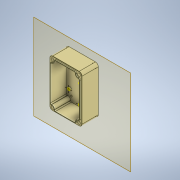
# Autodesk Inventor part: PinfoxBox
Saved by Autodesk Inventor 2021 (Build 250183000, 183)
## iProperties
Created: 2021-02-15
Part Number: PinfoxBox
Material: Polypropylene
Document SubType Name: Modeling
Designer: James
Density: 0.899 g/cm^3
Appearance: Smooth - Ash
Author: James
Autodesk Inventor part; units mm, degrees
ref_plane "YZ Plane" through (0, 0, 0) normal (1, 0, 0) x (0, 1, 0)
ref_plane "XZ Plane" through (0, 0, 0) normal (0, 1, 0) x (-1, 0, 0)
ref_plane "XY Plane" through (0, 0, 0) normal (0, 0, 1) x (1, 0, 0)
sketch "Drawing" plane through (0, 0, 0) normal (0, 0, 1) x (1, 0, 0)
  line L0 (-58.5227, 93.5052) -> (128.141, 93.5052) construction
  line L1 (128.141, 93.5052) -> (128.141, -71.3811) construction
  line L2 (128.141, -71.3811) -> (-58.5227, -71.3811) construction
  line L3 (-58.5227, -71.3811) -> (-58.5227, 93.5052) construction
  line L4 (-58.5227, 93.5052) -> (-58.5227, 50)
  line L5 (-54.9683, 50) -> (-54.9683, -50)
  line L6 (-58.5227, 50) -> (-54.9683, 50)
  line L7 (0, 0) -> (-54.9683, 0) construction
  line L8 (0, 0) -> (0, 93.5052) construction
  line L9 (0, 93.5052) -> (0, -71.3811)
  line L10 (-58.5227, 0) -> (128.141, 0)
  circle A0 centre (23, 22.25) radius 2.5
  circle A1 centre (23, 22.25) radius 1.5
  circle A2 centre (20, 35) radius 1.75
  dimension "d16" = 164.8863
  dimension "d20" = 3.5544
  dimension "d21" = 100
  dimension "d22" = 43.5052
  dimension "d48" = 5
  dimension "d49" = 1
  dimension "d50" = 3.5
  constraints: 14 end point, 5 point on line, 4 perpendicular, 3 centre point, 3 coincident, 1 horizontal, 1 midpoint, 1 vertical, 2 other
  measures "d16" distance of L2.end L0.start
  measures "d20" distance of L4.end L5.start
  measures "d21" distance of L5.start L5.end
  measures "d22" distance of L4.start L4.end
  measures "d48" diameter of A0
  measures "d49" radial gap between concentric circles of A0 A1
  measures "d50" diameter of A2
sketch "Sketch2" plane through (0, 0, 0) normal (0, 0, 1) x (1, 0, 0)
  line L0 (28, 50) -> (-28, 50)
  line L1 (-34, 44) -> (-34, -44)
  line L2 (-28, -50) -> (28, -50)
  line L3 (34, -44) -> (34, 44)
  line L4 (34, 50) -> (-34, -50) construction
  line L5 (-34, 50) -> (34, -50) construction
  arc A0 (-28, 50) -> (-34, 44) centre (-28, 44) ccw
  arc A1 (34, 44) -> (28, 50) centre (28, 44) ccw
  arc A2 (-34, -44) -> (-28, -50) centre (-28, -44) ccw
  arc A3 (28, -50) -> (34, -44) centre (28, -44) ccw
  line L6 (28.5085, 38) -> (28.519, 38)
  line L7 (28.0455, -38) -> (28.5, -38)
  line L8 (-58.5227, 0) -> (128.141, 0) projected
  line L9 (0, 0) -> (0, 93.5052) construction
  line L10 (0, 93.5052) -> (0, -71.3811) projected
  line L11 (22, 44) -> (22, 44.5)
  line L12 (30.5, 36) -> (30.5, -36)
  line L13 (22.0455, -44) -> (22.0455, -44.5)
  line L14 (-22.0163, -44.039) -> (-22.0163, -44.5)
  line L15 (-30.5, -36.039) -> (-30.5, 36)
  line L16 (-22, 44) -> (-22, 44.5)
  arc A4 (-28, 38) -> (-22, 44) centre (-28, 44) ccw
  arc A5 (22, 44) -> (28, 38) centre (28, 44) ccw
  arc A6 (28.0455, -38) -> (22.0455, -44) centre (28.0455, -44) ccw
  arc A7 (-22.0163, -44.039) -> (-28.0163, -38.039) centre (-28.0163, -44.039) ccw
  arc A8 (-22.0163, -44.5) -> (-20.0163, -46.5) centre (-20.0163, -44.5) ccw
  arc A9 (-30.5, -36.039) -> (-28.5, -38.039) centre (-28.5, -36.039) ccw
  arc A10 (20.0455, -46.5) -> (22.0455, -44.5) centre (20.0455, -44.5) ccw
  arc A11 (28.5, -38) -> (30.5, -36) centre (28.5, -36) ccw
  arc A12 (30.5, 36) -> (28.5, 38) centre (28.5, 36) ccw
  arc A13 (22, 44.5) -> (20, 46.5) centre (20, 44.5) ccw
  arc A14 (-28.5, 38) -> (-30.5, 36) centre (-28.5, 36) ccw
  arc A15 (-20, 46.5) -> (-22, 44.5) centre (-20, 44.5) ccw
  circle A16 centre (23, 22.25) radius 2.5
  circle A17 centre (23, 22.25) radius 1.5
  circle A18 centre (20, 35) radius 1.75
  circle A19 centre (-23, 22.25) radius 2.5
  circle A20 centre (-23, 22.25) radius 1.5
  circle A21 centre (-20, 35) radius 1.75
  circle A22 centre (23, -22.25) radius 2.5
  circle A23 centre (23, -22.25) radius 1.5
  circle A24 centre (20, -35) radius 1.75
  circle A25 centre (-20, -35) radius 1.75
  circle A26 centre (-23, -22.25) radius 2.5
  circle A27 centre (-23, -22.25) radius 1.5
  circle A28 centre (-28, 44) radius 2
  circle A29 centre (28, 44) radius 2
  circle A30 centre (-28, -44) radius 2
  circle A31 centre (28, -44) radius 2
  circle A32 centre (0, 40) radius 2.5
  circle A33 centre (0, 40) radius 1.5
  circle A34 centre (0, -40) radius 2.5
  circle A35 centre (0, -40) radius 1.5
  line L17 (-20.0163, -46.5) -> (20.0455, -46.5)
  line L18 (22, 44.4601) -> (22, 44)
  line L19 (-28, 38) -> (-28.5, 38)
  line L20 (-20, 46.5) -> (20, 46.5)
  line L21 (-28.5, -38.039) -> (-28.5, -38.039)
  line L22 (28.5, 38) -> (28, 38)
  line L23 (-28.493, -38.1054) -> (-28.493, -38.1054)
  line L24 (-28.5, -38.039) -> (-28.0163, -38.039)
  line L25 (23.05, 44) -> (23.05, 44.5)
  arc A36 (23.05, 44.5) -> (20, 47.55) centre (20, 44.5) ccw
  line L26 (20, 47.55) -> (-20, 47.55)
  arc A37 (-20, 47.55) -> (-23.05, 44.5) centre (-20, 44.5) ccw
  line L27 (-23.05, 44.5) -> (-23.05, 44)
  arc A38 (-28, 39.05) -> (-23.05, 44) centre (-28, 44) ccw
  line L28 (-28, 39.05) -> (-28.5, 39.05)
  arc A39 (-28.5, 39.05) -> (-31.55, 36) centre (-28.5, 36) ccw
  line L29 (-31.55, 36) -> (-31.55, -36.039)
  arc A40 (-31.55, -36.039) -> (-28.5, -39.089) centre (-28.5, -36.039) ccw
  line L30 (-28.5, -39.089) -> (-28.0163, -39.089)
  arc A41 (-23.0663, -44.039) -> (-28.0163, -39.089) centre (-28.0163, -44.039) ccw
  line L31 (-23.0663, -44.039) -> (-23.0663, -44.5)
  arc A42 (-23.0663, -44.5) -> (-20.0163, -47.55) centre (-20.0163, -44.5) ccw
  line L32 (-20.0163, -47.55) -> (20.0455, -47.55)
  arc A43 (20.0455, -47.55) -> (23.0955, -44.5) centre (20.0455, -44.5) ccw
  line L33 (23.0955, -44.5) -> (23.0955, -44)
  arc A44 (28.0455, -39.05) -> (23.0955, -44) centre (28.0455, -44) ccw
  line L34 (28.0455, -39.05) -> (28.5, -39.05)
  arc A45 (28.5, -39.05) -> (31.55, -36) centre (28.5, -36) ccw
  line L35 (31.55, -36) -> (31.55, 36)
  arc A46 (31.55, 36) -> (28.5, 39.05) centre (28.5, 36) ccw
  line L36 (28.5, 39.05) -> (28, 39.05)
  arc A47 (23.05, 44) -> (28, 39.05) centre (28, 44) ccw
  line L37 (-33.5, -44) -> (-33.5, 44)
  arc A48 (-28, 49.5) -> (-33.5, 44) centre (-28, 44) ccw
  line L38 (-28, 49.5) -> (28, 49.5)
  arc A49 (33.5, 44) -> (28, 49.5) centre (28, 44) ccw
  line L39 (33.5, 44) -> (33.5, -44)
  arc A50 (28, -49.5) -> (33.5, -44) centre (28, -44) ccw
  line L40 (28, -49.5) -> (-28, -49.5)
  arc A51 (-33.5, -44) -> (-28, -49.5) centre (-28, -44) ccw
  point P0 (-34, 38)
  point P1 (34, 38)
  point P2 (-34, -38)
  point P3 (34, -38)
  point P4 (22, 50)
  point P5 (22, -50)
  point P6 (-34, 46.5)
  point P7 (34, -46.5)
  dimension "OuterWidth" = 68
  dimension "OuterLength" = 100
  dimension "d26" = 6
  dimension "d27" = 6
  dimension "d29" = 6
  dimension "d34" = 6
  dimension "d36" = 2
  dimension "d37" = 6
  dimension "d38" = 6
  dimension "d39" = 6
  dimension "d40" = 6
  dimension "d41" = 11
  dimension "d42" = 27.75
  dimension "d43" = 5
  dimension "d44" = 1
  dimension "d45" = 3.5
  dimension "d46" = 15
  dimension "d47" = 14
  dimension "d52" = 4
  dimension "d53" = 5
  dimension "d54" = 1
  dimension "d55" = 10
  dimension "d56" = 3.5
  dimension "d57" = 3.5
  dimension "d58" = 3.5
  dimension "d59" = 3.5
  dimension "d60" = 6
  dimension "d61" = 6
  dimension "d62" = 6
  dimension "d63" = 6
  dimension "d67" = 1.05
  dimension "d68" = 1.05
  dimension "d86" = 0.5
  constraints: 76 end point, 69 point on circle, 52 centre point, 32 tangent, 23 point on line, 16 parallel, 10 symmetric about line, 2 equal radius, 2 midpoint, 2 perpendicular, 1 coincident, 1 horizontal, 43 other
  measures "OuterWidth" distance of L4.start L5.start
  measures "OuterLength" distance of L5.start L4.end
  measures "d26" distance from line of L1 point (-28, 44)
  measures "d27" distance from line of point (-28, 44) L0
  measures "d29" radius of A1
  measures "d34" radius of A4
  measures "d36" radius of A8
  measures "d37" distance from line of L0 A4.centre
  measures "d38" distance from line of L1 A4.centre
  measures "d39" distance from line of L3 A5.centre
  measures "d40" distance from line of L2 A6.centre
  measures "d41" distance from line of A16.centre L3
  measures "d42" distance from line of L0 A16.centre
  measures "d43" diameter of A16
  measures "d44" radial gap between concentric circles of A16 A17
  measures "d45" diameter of A18
  measures "d46" distance from line of L0 A18.centre
  measures "d47" distance from line of L3 A18.centre
  measures "d52" diameter of A28
  measures "d53" diameter of A32
  measures "d54" radial gap between concentric circles of A32 A33
  measures "d55" distance from line of L0 A32.centre
  measures "d56" distance between parallel lines of L0 L20
  measures "d57" distance between parallel lines of L15 L1
  measures "d58" distance between parallel lines of L3 L12
  measures "d59" distance between parallel lines of L2 L17
  measures "d60" radius of A6
  measures "d61" radius of A7
  measures "d62" radius of A5
  measures "d63" radius of A0
  measures "d67" distance between parallel lines of L20 L26
  measures "d68" radial gap between concentric circles of A7 A41
  measures "d86" distance between parallel lines of L1 L37
extrude "SideWalls" add sketch "Sketch2" along normal blind 35 contours A1 L3 L8 L39 A49 L38 L10 L0 | L10 L38 A48 L37 L8 L1 A0 L0 | L38 A49 L39 L8 L35 A46 L36 A47 L25 A36 L26 L10 | L10 L26 A37 L27 A38 L28 A39 L29 L8 L37 A48 L38 | L3 A3 L2 L10 L40 A50 L39 L8 | L26 A36 L25 A47 L36 A46 L35 L8 L12 A12 L6 L22 A5 L11 A13 L20 L10 | L10 L20 A15 L16 A4 L19 A14 L15 L8 L29 A39 L28 A38 L27 A37 L26 | L39 A50 L40 L10 L32 A43 L33 A44 L34 A45 L35 L8 | L8 L37 A51 L40 L10 L2 A2 L1 | L35 A45 L34 A44 L33 A43 L32 L10 L17 A10 L13 A6 L7 A11 L12 L8 | L8 L29 A40 L30 A41 L31 A42 L32 L10 L40 A51 L37 | L8 L15 A9 L24 A7 L14 A8 L17 L10 L32 A42 L31 A41 L30 A40 L29
extrude "GasketRingLower" add sketch "Sketch2" along normal blind 36.85 contours L26 A36 L25 A47 L36 A46 L35 L8 L12 A12 L6 L22 A5 L11 A13 L20 L10 | L10 L20 A15 L16 A4 L19 A14 L15 L8 L29 A39 L28 A38 L27 A37 L26 | L35 A45 L34 A44 L33 A43 L32 L10 L17 A10 L13 A6 L7 A11 L12 L8 | L8 L15 A9 L24 A7 L14 A8 L17 L10 L32 A42 L31 A41 L30 A40 L29
extrude "Bottom" add sketch "Sketch2" along normal blind 2.8 contours A1 L3 L8 L39 A49 L38 L10 L0 | L10 L38 A48 L37 L8 L1 A0 L0 | L38 A49 L39 L8 L35 A46 L36 A47 L25 A36 L26 L10 | L10 L26 A37 L27 A38 L28 A39 L29 L8 L37 A48 L38 | L3 A3 L2 L10 L40 A50 L39 L8 | L26 A36 L25 A47 L36 A46 L35 L8 L12 A12 L6 L22 A5 L11 A13 L20 L10 | L10 L20 A15 L16 A4 L19 A14 L15 L8 L29 A39 L28 A38 L27 A37 L26 | L39 A50 L40 L10 L32 A43 L33 A44 L34 A45 L35 L8 | L8 L37 A51 L40 L10 L2 A2 L1 | L20 A13 L11 A5 L22 A12 L6 L12 L8 L10 A32 | L10 A32 L8 L15 A14 L19 A4 L16 A15 L20 | L35 A45 L34 A44 L33 A43 L32 L10 L17 A10 L13 A6 L7 A11 L12 L8 | L8 L29 A40 L30 A41 L31 A42 L32 L10 L40 A51 L37 | A32 L10 A33 | L10 A33 A32 | L12 A11 L7 A6 L13 A10 L17 L10 A34 L8 | L8 L15 A9 L24 A7 L14 A8 L17 L10 L32 A42 L31 A41 L30 A40 L29 | A33 L10 | L10 A33 | L10 A34 L17 A8 L14 A7 L24 A9 L15 L8 | A34 L10 A35 | L10 A35 A34 | A35 L10 | L10 A35 | A16 | A17 | A18 | A19 | A20 | A21 | A22 | A23 | A24 | A25 | A26 | A27 | A28 | A29 | A30 | A31
extrude "PEMStuds" add sketch "Sketch2" along normal blind 6 contours A32 L10 A33 | L10 A33 A32 | A33 L10 | L10 A33 | A34 L10 A35 | L10 A35 A34 | A35 L10 | L10 A35 | A16 | A17 | A19 | A20 | A22 | A23 | A26 | A27
extrude "SmallerSupports" add sketch "Sketch2" along normal blind 4 contours A18 | A21 | A24 | A25
sketch "Sketch4" plane through (-23, -22.25, 6) normal (0, 0, 1) x (1, 0, 0)
  circle A0 centre (23, -17.75) radius 2.5 projected
  circle A1 centre (46, 0) radius 2.5 projected
  circle A2 centre (23, 62.25) radius 2.5 projected
  circle A3 centre (0, 0) radius 2.5 projected
  circle A4 centre (46, 44.5) radius 2.5 projected
  circle A5 centre (-5, -21.75) radius 2 projected
  circle A6 centre (51, -21.75) radius 2 projected
  circle A7 centre (-5, 66.25) radius 2 projected
  circle A8 centre (51, 66.25) radius 2 projected
  point P0 (23, 22.25)
  point P1 (0, 44.5)
  point P2 (0, 44.5)
  constraints: 10 coincident
hole "PEMStudHoles" at (0, -40, 6) at (23, -22.25, 6) at (0, 40, 6) at (-23, -22.25, 6) at (23, 22.25, 6) at (-23, 22.25, 6) direction (0, 0, -1) diameter 3 depth 4
hole "Hole2" at (28, 44, 6) at (-28, 44, 6) at (-28, -44, 6) at (28, -44, 6) direction (0, 0, -1) diameter 6 end through all both
ref_plane "Work Plane2" through (-32.2426, 48.2426, 35) normal (0, 0, 1) x (1, 0, 0)
sketch "Sketch6" plane through (-32.2426, 48.2426, 35) normal (0, 0, 1) x (1, 0, 0)
  line L0 (-1.2574, -92.2426) -> (-1.2574, -4.2426) projected
  arc A0 (4.2426, 1.2574) -> (-1.2574, -4.2426) centre (4.2426, -4.2426) ccw projected
  line L1 (4.2426, 1.2574) -> (60.2426, 1.2574) projected
  arc A1 (65.7426, -4.2426) -> (60.2426, 1.2574) centre (60.2426, -4.2426) ccw projected
  line L2 (65.7426, -4.2426) -> (65.7426, -92.2426) projected
  arc A2 (60.2426, -97.7426) -> (65.7426, -92.2426) centre (60.2426, -92.2426) ccw projected
  line L3 (60.2426, -97.7426) -> (4.2426, -97.7426) projected
  arc A3 (-1.2574, -92.2426) -> (4.2426, -97.7426) centre (4.2426, -92.2426) ccw projected
  line L4 (-1.7574, -4.2426) -> (-1.7574, -92.2426)
  arc A4 (-1.7574, -92.2426) -> (4.2426, -98.2426) centre (4.2426, -92.2426) ccw
  line L5 (4.2426, -98.2426) -> (60.2426, -98.2426)
  arc A5 (60.2426, -98.2426) -> (66.2426, -92.2426) centre (60.2426, -92.2426) ccw
  line L6 (66.2426, -92.2426) -> (66.2426, -4.2426)
  arc A6 (66.2426, -4.2426) -> (60.2426, 1.7574) centre (60.2426, -4.2426) ccw
  line L7 (60.2426, 1.7574) -> (4.2426, 1.7574)
  arc A7 (4.2426, 1.7574) -> (-1.7574, -4.2426) centre (4.2426, -4.2426) ccw
  line L8 (4.2426, 1.2574) -> (60.2426, 1.2574)
  arc A8 (65.7426, -4.2426) -> (60.2426, 1.2574) centre (60.2426, -4.2426) ccw
  line L9 (65.7426, -4.2426) -> (65.7426, -92.2426)
  arc A9 (60.2426, -97.7426) -> (65.7426, -92.2426) centre (60.2426, -92.2426) ccw
  line L10 (60.2426, -97.7426) -> (4.2426, -97.7426)
  arc A10 (-1.2574, -92.2426) -> (4.2426, -97.7426) centre (4.2426, -92.2426) ccw
  line L11 (-1.2574, -92.2426) -> (-1.2574, -4.2426)
  arc A11 (4.2426, 1.2574) -> (-1.2574, -4.2426) centre (4.2426, -4.2426) ccw
  point P0 (32.2426, -48.2426)
  dimension "d97" = 0.5
  dimension "d98" = 0.5
  constraints: 16 end point, 16 point on circle, 8 centre point, 14 other
  measures "d97" distance between parallel lines of L0 L4
  measures "d98" distance between parallel lines of L7 L8
extrude "Extrusion8" cut sketch "Sketch6" against normal blind 0.5
equation "\"d16\" = 280.458 * ImageScale"
equation "\"d20\" = 6.04577 * ImageScale"
equation "\"d21\" = 170.092 * ImageScale"
equation "\"d22\" = 73.9989 * ImageScale"
equation "\"d26\" = OuterFillet"
equation "\"d27\" = OuterFillet"
equation "\"d29\" = OuterFillet"
equation "\"d37\" = OuterFillet"
equation "\"d38\" = OuterFillet"
equation "\"d39\" = OuterFillet"
equation "\"d40\" = OuterFillet"
equation "\"ImageScale\" = 0.587917"
equation "\"WallThickness\" = 3.5"
equation "\"OuterFillet\" = 6"
body "Solid1"
